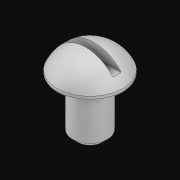
# Autodesk Inventor part: AScrew .250
Saved by Autodesk Inventor 2021 (Build 250183000, 183)
## iProperties
Created: 2020-07-03
Part Number: AScrew .250
Material: VEX Aluminum Alloy 5052-H32
Document SubType Name: Modeling
Designer: yuany
Density: 2.68277 g/cm^3
Appearance: Standoffs
Author: yuany
Autodesk Inventor part; units mm, degrees
ref_plane "YZ Plane" through (0, 0, 0) normal (1, 0, 0) x (0, 1, 0)
ref_plane "XZ Plane" through (0, 0, 0) normal (0, 1, 0) x (-1, 0, 0)
ref_plane "XY Plane" through (0, 0, 0) normal (0, 0, 1) x (1, 0, 0)
sketch "Sketch1" plane through (0, 0, 0) normal (0, 1, 0) x (-1, 0, 0)
  circle A0 centre (0, 0) radius 2.0828
  dimension "d4" = 4.1656
  constraints: 1 centre point, 1 coincident
  measures "d4" diameter of A0
extrude "Body" add sketch "Sketch1" along normal blind 6.35
sketch "Sketch2" plane through (0, 0, 0) normal (1, 0, 0) x (0, 1, 0)
  line L0 (6.35, -2.0828) -> (6.35, 2.0828) projected
  line L1 (6.35, 0) -> (6.35, -3.7846)
  line L2 (6.8072, 0) -> (6.35, 0)
  line L3 (6.8072, 0) -> (6.8072, -3.937)
  arc A0 (6.8072, -3.937) -> (9.3815, 0) centre (5.0838, 0) ccw
  line L4 (6.5024, -3.937) -> (6.8072, -3.937)
  line L5 (6.8072, 0) -> (9.3815, 0)
  arc A1 (6.35, -3.7846) -> (6.5024, -3.937) centre (6.5024, -3.7846) ccw
  point P0 (0, 0)
  point P1 (6.35, -3.937)
  dimension "d5" = 3.937
  dimension "d13" = 0.4572
  dimension "d57" = 3.937
  dimension "d58" = 4.2977
  dimension "d59" = 0
  dimension "d67" = 0.1524
  constraints: 10 end point, 4 point on circle, 4 point on line, 2 centre point, 2 horizontal, 2 tangent, 1 midpoint, 1 vertical
  measures "d5" distance of L1.start point (6.35, -3.937)
  measures "d13" distance of L2.start L1.start
  measures "d57" distance of L2.start L3.end
  measures "d58" radius of A0
  measures "d59" distance from line of L2 A0.centre
  measures "d67" radius of A1
revolve "Head" add sketch "Sketch2" angle 360 about axis through (0, 6.8072, 0) along (0, -1, 0)
feature "Thread" [suppressed]
sketch "Sketch6" plane through (0, 0, 0) normal (0, 0, 1) x (1, 0, 0)
  line L0 (0, 0) -> (-1.4859, 0)
  line L1 (2.0828, 0) -> (-2.0828, 0) projected
  line L2 (-1.4859, 0) -> (-2.4948, 1.0089)
  line L3 (-2.4948, 1.0089) -> (-2.9651, -1.2188)
  line L4 (-2.9651, -1.2188) -> (-1.4859, -1.2188)
  line L5 (-2.0828, 0) -> (-2.0828, 6.35) projected
  line L6 (-1.4859, -1.2188) -> (-1.4859, 0)
  line L7 (0, -2.9358) -> (0, 9.083) projected
  point P0 (-2.0828, 0.5969)
  dimension "d49" = 1.4859
  dimension "d50" = 135
  constraints: 10 end point, 1 perpendicular, 1 point on line, 1 vertical
  measures "d49" distance from line of L0.start L6
  measures "d50" angle of L2 L6
revolve "Tapered End" cut sketch "Sketch6" angle 360 about axis through (0, -10, 0) along (0, 1, 0)
sketch "Sketch7" plane through (0, 0, 0) normal (1, 0, 0) x (0, 1, 0)
  line L0 (31.75, 4.3688) -> (31.75, -4.3688) projected
  line L1 (7.874, 0.4953) -> (7.874, -0.4953)
  line L2 (7.874, 0.4953) -> (9.8806, 0.4953)
  line L3 (9.8806, 0.4953) -> (9.8806, -0.4953)
  line L4 (9.8806, -0.4953) -> (7.874, -0.4953)
  point P0 (0, 0)
  dimension "d61" = 0.9906
  dimension "d62" = 0.4953
  dimension "d65" = 7.874
  dimension "d66" = 2.0066
  constraints: 8 end point, 1 horizontal, 1 parallel, 1 perpendicular, 1 vertical
  measures "d61" distance of L2.end L3.end
  measures "d62" distance from line of L2 point (0, 0)
  measures "d65" distance from line of point (0, 0) L1
  measures "d66" distance of L1.start L2.end
extrude "Flathead" cut sketch "Sketch7" against normal mid plane 12.7
sketch "Sketch5" plane through (0, 0, 0) normal (1, 0, 0) x (0, 1, 0)
  line L0 (0.0745, -1.5621) -> (-0.2261, -2.0828)
  line L1 (-0.2261, -2.0828) -> (-0.3253, -2.0828)
  line L2 (-0.3253, -2.0828) -> (-0.626, -1.5621)
  line L3 (0.0686, -2.0828) -> (-0.7252, -2.0828) construction
  line L4 (-0.626, -1.5621) -> (0.0745, -1.5621)
  line L5 (0, -1.5621) -> (31.75, -1.5621)
  point P0 (0, 0)
  dimension "d32" = 60
  dimension "a" = 0.0992
  dimension "d46" = 0.7937
  dimension "d54" = 0.0686
  dimension "d55" = 0.5207
  dimension "d56" = 0.0992
  constraints: 12 end point, 2 collinear, 1 equal length, 1 horizontal
  measures "d32" angle of L0 L2
  measures "a" distance of L0.end L1.end
  measures "d46" distance of L3.start L3.end
  measures "d54" horizontal distance of L3.start L5.start
  measures "d55" distance between parallel lines of L1 L4
  measures "d56" horizontal distance of L2.end L3.end
equation "\"d56\" = a"
body "Solid1"
